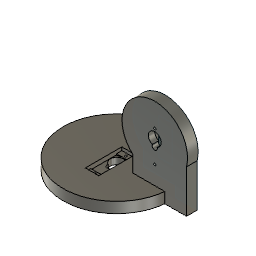
Base Link (Autodesk Fusion 360 design; units mm, degrees)
part number: 2026-08-19-17-00-12-411
Autodesk Fusion 360 part; units mm, degrees
note: some values were not read from the file. Chosen so that the rebuilt part matches the saved one: a direction; how an offset face is resized. Set by a fixed rule: which sketch regions a step uses.
sketch "Sketch1" plane through (0, 0, 0) normal (0, 0, 1) x (1, 0, 0)
  circle A0 centre (0, 0) radius 50
  dimension "d1" = 100
  constraint coincident A0.centre origin
  measures "d1" diameter of A0
extrude "Extrude1" add sketch "Sketch1" along normal blind 10
sketch "Sketch2" plane through (0, 0, 10) normal (0, 0, 1) x (-1, 0, 0)
  circle A0 centre (0, 0) radius 50
  line L0 (-6.25, -11) -> (6.25, -11)
  line L1 (6.25, -11) -> (6.25, 23)
  line L2 (6.25, 23) -> (-6.25, 23)
  line L3 (-6.25, 23) -> (-6.25, -11)
  line L4 (-6.25, -11) -> (6.25, 23) construction
  line L5 (6.25, -11) -> (-6.25, 23) construction
  line L6 (6.25, -6) -> (-6.25, -6)
  line L7 (6.25, 18) -> (-6.25, 18)
  point P0 (0, 6)
  point P1 (0, 6)
  dimension "d4" = 6
  dimension "d5" = 12.5
  dimension "d6" = 34
  dimension "d7" = 5
  dimension "d8" = 5
  constraint coincident A0.centre origin
  constraint horizontal L0
  constraint perpendicular L0 L1
  constraint parallel L0 L2
  constraint parallel L1 L3
  constraint coincident L4 P1
  constraint coincident L5 P1
  constraint coincident P1 P0
  constraint coincident L1 L6.start
  constraint coincident L3 L6.end
  constraint perpendicular L3 L6
  constraint coincident L1 L7.start
  constraint coincident L3 L7.end
  constraint perpendicular L3 L7
  measures "d4" distance of A0.centre P1
  measures "d5" distance of L1.end L2.end
  measures "d6" distance of L0.end L1.end
  measures "d7" distance of L0 L6
  measures "d8" distance of L2 L7
extrude "Extrude2" cut sketch "Sketch2" against normal blind 3 contours L0 L1 L3 L6 | L1 L3 L6 L7 | L1 L2 L3 L7
sketch "Sketch3" plane through (0, 0, 7) normal (0, 0, 1) x (-1, 0, 0)
  line L0 (-6.25, 23) -> (-6.25, -11)
  line L1 (-6.25, -11) -> (6.25, -11)
  line L2 (6.25, -11) -> (6.25, 23)
  line L3 (6.25, 23) -> (-6.25, 23)
  line L4 (6.25, -6) -> (-6.25, -6)
  line L5 (6.25, 18) -> (-6.25, 18)
  dimension "d11" = 5
  dimension "d12" = 5
  constraint coincident L2 L4.start
  constraint coincident L0 L4.end
  constraint perpendicular L0 L4
  constraint coincident L2 L5.start
  constraint coincident L0 L5.end
  constraint perpendicular L0 L5
  measures "d11" distance of L1 L4
  measures "d12" distance of L3 L5
extrude "Extrude3" cut sketch "Sketch3" against normal blind 1 contours L0 L2 L4 L5
sketch "Sketch4" plane through (0, 0, 6) normal (0, 0, 1) x (-1, 0, 0)
  line L0 (6.25, -6) -> (6.25, 18)
  line L1 (6.25, 18) -> (-6.25, 18)
  line L2 (-6.25, 18) -> (-6.25, -6)
  line L3 (-6.25, -6) -> (6.25, -6)
  circle A0 centre (0, 0) radius 6
  circle A1 centre (0, 6.5) radius 2.5
  dimension "d15" = 12
  dimension "d16" = 5
  dimension "d17" = 6.5
  constraint tangent L3 A0
  measures "d15" diameter of A0
  measures "d16" diameter of A1
  measures "d17" distance of A0.centre A1.centre
extrude "Extrude4" cut sketch "Sketch4" against normal blind 6 contours A0 A1 | A0 A1 | A0 A1
sketch "Sketch5" plane through (0, 0, 7) normal (0, 0, 1) x (-1, 0, 0)
  line L0 (-6.25, 18) -> (6.25, 18)
  line L1 (6.25, 18) -> (6.25, 23)
  line L2 (6.25, 23) -> (-6.25, 23)
  line L3 (-6.25, 23) -> (-6.25, 18)
  circle A0 centre (0, 20.5) radius 1.25
  dimension "d20" = 2.5
  dimension "d21" = 2.5
  measures "d20" diameter of A0
  measures "d21" distance of L2 A0.centre
sketch "Sketch6" plane through (0, 0, 7) normal (0, 0, 1) x (-1, 0, 0)
  line L0 (6.25, -6) -> (-6.25, -6)
  line L1 (-6.25, -6) -> (-6.25, -11)
  line L2 (-6.25, -11) -> (6.25, -11)
  line L3 (6.25, -11) -> (6.25, -6)
  circle A0 centre (0, -8.5) radius 1.25
  dimension "d22" = 2.5
  dimension "d23" = 2.5
  measures "d22" diameter of A0
  measures "d23" distance of L0 A0.centre
extrude "Extrude5" cut sketch "Sketch6" against normal through all contours A0
extrude "Extrude6" cut sketch "Sketch5" against normal through all contours A0
thread "Thread1" "ISO Metric profile 2.5 M2.5x0.45 M2.5x0.45 6H" major diameter 2.58 minor diameter 2.0755 pitch 0.45 angle 60 resizes the face on face at (-1.2438, -20.3755, 4.6667)
thread "Thread2" "ISO Metric profile 2.5 M2.5x0.45 M2.5x0.45 6H" major diameter 2.58 minor diameter 2.0755 pitch 0.45 angle 60 resizes the face on face at (-1.2438, 8.6245, 4.6667)
sketch "Sketch7" plane through (0, 0, 0) normal (0, 1, 0) x (1, 0, 0)
  line L0 (20, 0) -> (70, 0)
  line L1 (70, 0) -> (70, -40)
  arc A0 (20, -25) -> (70, -40) centre (40.4442, -47.6861) ccw
  line L2 (20, -25) -> (20, 0)
  dimension "d30" = 50
  dimension "d31" = 40
  dimension "d32" = 20
  constraint horizontal L0
  constraint perpendicular L0 L1
  constraint perpendicular L0 L2
  measures "d30" distance of L0.start L0.end
  measures "d31" distance of L0.end L1.end
  measures "d32" distance of origin L0.start
extrude "Extrude7" add sketch "Sketch7" along normal mid plane 10
sketch "Sketch8" plane through (0, 5, 0) normal (0, 1, 0) x (-1, 0, 0)
  line L0 (-49.7494, 10) -> (-20, 10)
  line L1 (-20, 10) -> (-20, 25)
  arc A0 (-20, 25) -> (-70, 40) centre (-40.4442, 47.6861) ccw
  line L2 (-70, 40) -> (-70, 0)
  line L3 (-70, 0) -> (-49.7494, 0)
  line L4 (-49.7494, 0) -> (-49.7494, 10)
  line L5 (-34.1942, 24.6861) -> (-46.6942, 24.6861)
  line L6 (-46.6942, 24.6861) -> (-46.6942, 58.6861)
  line L7 (-46.6942, 58.6861) -> (-34.1942, 58.6861)
  line L8 (-34.1942, 58.6861) -> (-34.1942, 24.6861)
  line L9 (-34.1942, 24.6861) -> (-46.6942, 58.6861) construction
  line L10 (-46.6942, 24.6861) -> (-34.1942, 58.6861) construction
  point P0 (-40.4442, 47.6861)
  point P1 (-40.4442, 41.6861)
  point P2 (-40.4442, 41.6861)
  dimension "d35" = 6
  dimension "d36" = 12.5
  dimension "d37" = 34
  constraint coincident P0 A0.centre
  constraint horizontal L5
  constraint perpendicular L5 L6
  constraint parallel L5 L7
  constraint parallel L6 L8
  constraint coincident L9 P2
  constraint coincident L10 P2
  constraint coincident P2 P1
  measures "d35" distance of P0 P2
  measures "d36" distance of L6.end L7.end
  measures "d37" distance of L5.end L6.end
extrude "Extrude8" cut sketch "Sketch8" against normal blind 3 contours L5 L6 L7 L8
sketch "Sketch9" plane through (0, 2, 0) normal (0, 1, 0) x (-1, 0, 0)
  line L0 (-34.1942, 58.6861) -> (-46.6942, 58.6861)
  line L1 (-46.6942, 58.6861) -> (-46.6942, 24.6861)
  line L2 (-46.6942, 24.6861) -> (-34.1942, 24.6861)
  line L3 (-34.1942, 24.6861) -> (-34.1942, 58.6861)
  line L4 (-46.6942, 53.6861) -> (-34.1942, 53.6861)
  line L5 (-46.6942, 29.6861) -> (-34.1942, 29.6861)
  dimension "d40" = 5
  dimension "d41" = 5
  constraint coincident L1 L4.start
  constraint coincident L3 L4.end
  constraint perpendicular L3 L4
  constraint coincident L1 L5.start
  constraint coincident L3 L5.end
  constraint perpendicular L3 L5
  measures "d40" distance of L0 L4
  measures "d41" distance of L2 L5
extrude "Extrude9" cut sketch "Sketch9" against normal blind 1 contours L1 L3 L4 L5
sketch "Sketch10" plane through (0, 1, 0) normal (0, 1, 0) x (-1, 0, 0)
  line L0 (-46.6942, 53.6861) -> (-46.6942, 29.6861)
  line L1 (-46.6942, 29.6861) -> (-34.1942, 29.6861)
  line L2 (-34.1942, 29.6861) -> (-34.1942, 53.6861)
  line L3 (-34.1942, 53.6861) -> (-46.6942, 53.6861)
  circle A0 centre (-40.4442, 47.6861) radius 6
  circle A1 centre (-40.4442, 41.1861) radius 2.5
  dimension "d44" = 12
  dimension "d45" = 5
  dimension "d46" = 6.5
  constraint tangent L3 A0
  measures "d44" diameter of A0
  measures "d45" diameter of A1
  measures "d46" distance of A0.centre A1.centre
extrude "Extrude10" cut sketch "Sketch10" against normal blind 6 contours A0 A1 | A0 A1 | A0 A1
sketch "Sketch11" plane through (0, 2, 0) normal (0, 1, 0) x (-1, 0, 0)
  line L0 (-34.1942, 29.6861) -> (-46.6942, 29.6861)
  line L1 (-46.6942, 29.6861) -> (-46.6942, 24.6861)
  line L2 (-46.6942, 24.6861) -> (-34.1942, 24.6861)
  line L3 (-34.1942, 24.6861) -> (-34.1942, 29.6861)
  circle A0 centre (-40.4442, 27.1861) radius 1.25
  dimension "d49" = 2.5
  dimension "d50" = 2.5
  measures "d49" diameter of A0
  measures "d50" distance of L2 A0.centre
sketch "Sketch12" plane through (0, 2, 0) normal (0, 1, 0) x (-1, 0, 0)
  line L0 (-46.6942, 53.6861) -> (-34.1942, 53.6861)
  line L1 (-34.1942, 53.6861) -> (-34.1942, 58.6861)
  line L2 (-34.1942, 58.6861) -> (-46.6942, 58.6861)
  line L3 (-46.6942, 58.6861) -> (-46.6942, 53.6861)
  circle A0 centre (-40.4442, 56.1861) radius 1.25
  dimension "d51" = 2.5
  dimension "d52" = 2.5
  measures "d51" diameter of A0
  measures "d52" distance of L0 A0.centre
extrude "Extrude11" cut sketch "Sketch12" against normal through all contours A0
extrude "Extrude12" cut sketch "Sketch11" against normal through all contours A0
thread "Thread3" "ISO Metric profile 2.5 M2.5x0.45 M2.5x0.45 6H" major diameter 2.58 minor diameter 2.0755 pitch 0.45 angle 60 resizes the face on face at (39.2004, -0.3333, 27.0616) on face at (41.596, -2.6667, 55.7005)
sketch "Sketch13" plane through (0, 5, 0) normal (0, 1, 0) x (-1, 0, 0)
  line L0 (-46.6942, 24.6861) -> (-46.6942, 58.6861)
  line L1 (-46.6942, 58.6861) -> (-34.1942, 58.6861)
  line L2 (-34.1942, 58.6861) -> (-34.1942, 24.6861)
  line L3 (-34.1942, 24.6861) -> (-46.6942, 24.6861)
  line L4 (-49.7494, 10) -> (-20, 10)
  line L5 (-20, 10) -> (-20, 25)
  arc A0 (-20, 25) -> (-70, 40) centre (-40.4442, 47.6861) ccw
  line L6 (-70, 40) -> (-70, 0)
  line L7 (-70, 0) -> (-49.7494, 0)
  line L8 (-49.7494, 0) -> (-49.7494, 10)
